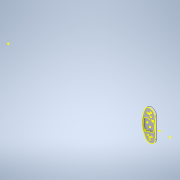
# Autodesk Inventor part: クランク
Saved by Autodesk Inventor 2022.2 (Build 262287000, 287)
## iProperties
Created: 2021-12-23
Part Number: クランク
Material: Generic
Document SubType Name: Modeling
Designer: acps
Density: 1 g/cm^3
Appearance: Default
Author: acps
Autodesk Inventor part; units mm, degrees
ref_plane "YZ Plane" through (0, 0, 0) normal (1, 0, 0) x (0, 1, 0)
ref_plane "XZ Plane" through (0, 0, 0) normal (0, 1, 0) x (-1, 0, 0)
ref_plane "XY Plane" through (0, 0, 0) normal (0, 0, 1) x (1, 0, 0)
sketch "Sketch1" plane through (0, 0, 0) normal (0, 0, 1) x (1, 0, 0)
  line L0 (-15.8764, 0) -> (-29.8764, 0)
  line L1 (-15.8764, 0) -> (-7.3764, 0)
  line L2 (-25.9706, 16.9706) -> (-25.9706, -16.9706) construction
  line L3 (-7.9706, -16.9706) -> (-7.9706, 16.9706) construction
  arc A0 (-7.9706, 16.9706) -> (-7.9926, 17.6) centre (-16.9706, 16.9706) ccw construction
  arc A1 (-25.9706, -16.9706) -> (-25.0651, -20.9049) centre (-16.9706, -16.9706) ccw construction
  arc A2 (-25.0651, 20.9049) -> (-25.0651, -20.9049) centre (17.9444, 0) ccw
  arc A3 (-7.9926, -17.6) -> (-7.9926, 17.6) centre (-259.0334, 0) ccw
  arc A4 (-25.0651, 20.9049) -> (-25.9706, 16.9706) centre (-16.9706, 16.9706) ccw construction
  arc A5 (-25.0651, -20.9049) -> (-7.9926, -17.6) centre (-16.9706, -16.9706) ccw
  arc A6 (-7.9926, 17.6) -> (-25.0651, 20.9049) centre (-16.9706, 16.9706) ccw
  arc A7 (-7.9926, -17.6) -> (-7.9706, -16.9706) centre (-16.9706, -16.9706) ccw construction
  line L4 (-16.9706, -20.5501) -> (-20.0706, -15.1808) construction
  line L5 (-20.0706, -15.1808) -> (-13.8706, -15.1808) construction
  line L6 (-13.8706, -15.1808) -> (-16.9706, -20.5501) construction
  circle A8 centre (-20.0706, -15.1808) radius 1.25
  circle A9 centre (-13.8706, -15.1808) radius 1.25
  circle A10 centre (-16.9706, -20.5501) radius 1.25
  line L7 (0, 0) -> (-43.2466, 0) construction
  line L8 (-15.1808, 20.0706) -> (-15.1808, 13.8706) construction
  line L9 (-15.1808, 13.8706) -> (-20.5501, 16.9706) construction
  line L10 (-20.5501, 16.9706) -> (-15.1808, 20.0706) construction
  circle A11 centre (-15.1808, 13.8706) radius 1.25
  circle A12 centre (-20.5501, 16.9706) radius 1.25
  circle A13 centre (-15.1808, 20.0706) radius 1.25
  line L11 (-16.9706, 16.9706) -> (0, 0) construction
  line L12 (-16.9706, -16.9706) -> (0, 0) construction
  point P0 (-29.8764, 0)
  point P1 (-7.3764, 0)
  dimension "d11" = 9
  dimension "d14" = 2.5
  dimension "d15" = 2.5
  dimension "d16" = 2.5
  dimension "d17" = 6.2
  dimension "d19" = 2.5
  dimension "d20" = 2.5
  dimension "d21" = 2.5
  dimension "d22" = 6.2
  dimension "d23" = 24
  dimension "d24" = 45
  dimension "d25" = 24
  dimension "d26" = 45
  dimension "d27" = 14
  dimension "d28" = 8.5
  constraints: 24 end point, 22 point on circle, 14 centre point, 8 coincident, 8 tangent, 4 horizontal, 2 point on line, 2 vertical, 24 other
  measures "d11" radius of A1
  measures "d14" diameter of A8
  measures "d15" diameter of A9
  measures "d16" diameter of A10
  measures "d17" distance of L5.end L4.end
  measures "d19" diameter of A11
  measures "d20" diameter of A12
  measures "d21" diameter of A13
  measures "d22" distance of L9.end L8.end
  measures "d23" distance of L11.start L7.start
  measures "d24" angle of L7 L11
  measures "d25" distance of L12.start L7.start
  measures "d26" angle of L7 L12
  measures "d27" distance of point (-29.876, 0) L0.start
  measures "d28" distance of point (-7.376, 0) L0.start
extrude "Extrusion1" add sketch "Sketch1" along normal blind 3
sketch "Sketch2" plane through (0, 0, 3) normal (0, 0, 1) x (1, 0, 0)
  arc A0 (-25.0651, 20.9049) -> (-25.0651, -20.9049) centre (17.9444, 0) ccw projected
  arc A1 (-25.0651, -20.9049) -> (-7.9926, -17.6) centre (-16.9706, -16.9706) ccw projected
  arc A2 (-7.9926, -17.6) -> (-7.9926, 17.6) centre (-259.0334, 0) ccw projected
  arc A3 (-7.9926, 17.6) -> (-25.0651, 20.9049) centre (-16.9706, 16.9706) ccw projected
  circle A4 centre (-16.9706, -20.5501) radius 1.25 projected
  circle A5 centre (-13.8706, -15.1808) radius 1.25 projected
  circle A6 centre (-20.0706, -15.1808) radius 1.25 projected
  circle A7 centre (-15.1808, 13.8706) radius 1.25 projected
  circle A8 centre (-15.1808, 20.0706) radius 1.25 projected
  circle A9 centre (-20.5501, 16.9706) radius 1.25 projected
  arc A10 (-23.2663, 20.0306) -> (-23.2663, -20.0306) centre (17.9444, 0) ccw
  arc A11 (-9.9877, 17.4601) -> (-23.2663, 20.0306) centre (-16.9706, 16.9706) ccw
  arc A12 (-9.9877, -17.4601) -> (-9.9877, 17.4601) centre (-259.0334, 0) ccw
  arc A13 (-23.2663, -20.0306) -> (-9.9877, -17.4601) centre (-16.9706, -16.9706) ccw
  circle A14 centre (-15.1808, 13.8706) radius 4.25
  circle A15 centre (-16.9706, 16.9706) radius 7.8296
  circle A16 centre (-16.9706, -16.9706) radius 7.8296
  line L0 (-9.7642, 13.9095) -> (10.6825, 13.9095)
  point P0 (0, 0)
  point P1 (-24.7881, -16.5371)
  point P2 (-9.7642, -13.9095)
  point P3 (-24.7881, 16.5371)
  dimension "d33" = 15.6591
  dimension "d31" = 2
  dimension "d32" = 3
  dimension "d34" = 15.6591
  constraints: 9 point on circle, 6 centre point, 2 coincident, 2 end point, 1 horizontal, 7 other
  measures "d31" radial gap between concentric circles of A0 A10
  measures "d32" radial gap between concentric circles of A7 A14
  measures "d34" diameter of A16
extrude "Extrusion2" cut sketch "Sketch2" against normal blind 2 contours A15 A12 A16 A10
fillet "Fillet1" radius 7 2 edges at (-24.7881, 16.5371, 2) (-9.7642, -13.9095, 2)
fillet "Fillet2" radius 2 2 edges at (-9.7642, 13.9095, 2) (-24.7881, -16.5371, 2)
sketch "Sketch3" plane through (0, 0, 3) normal (0, 0, 1) x (1, 0, 0)
  arc A0 (-18.9853, 9.4046) -> (-12.6387, 10.4485) centre (-16.9706, 16.9706) ccw projected
  arc A1 (-9.5334, 8.8534) -> (-12.6387, 10.4485) centre (-11.5322, 8.7825) ccw projected
  arc A2 (-9.3862, -2.2146) -> (-9.5334, 8.8534) centre (-259.0334, 0) ccw projected
  arc A3 (-16.6619, -9.1471) -> (-9.3862, -2.2146) centre (-16.386, -2.1525) ccw projected
  arc A4 (-16.6619, -9.1471) -> (-23.006, -11.983) centre (-16.9706, -16.9706) ccw projected
  arc A5 (-26.4871, -11.1978) -> (-23.006, -11.983) centre (-24.5477, -10.709) ccw projected
  arc A6 (-27.7703, 3.1165) -> (-26.4871, -11.1978) centre (17.9444, 0) ccw projected
  arc A7 (-18.9853, 9.4046) -> (-27.7703, 3.1165) centre (-20.7865, 2.6404) ccw projected
  arc A8 (-25.0651, 20.9049) -> (-25.0651, -20.9049) centre (17.9444, 0) ccw projected
  arc A9 (-25.0651, -20.9049) -> (-7.9926, -17.6) centre (-16.9706, -16.9706) ccw projected
  arc A10 (-7.9926, -17.6) -> (-7.9926, 17.6) centre (-259.0334, 0) ccw projected
  arc A11 (-7.9926, 17.6) -> (-25.0651, 20.9049) centre (-16.9706, 16.9706) ccw projected
  circle A12 centre (-16.9706, -20.5501) radius 1.25 projected
  circle A13 centre (-13.8706, -15.1808) radius 1.25 projected
  circle A14 centre (-20.0706, -15.1808) radius 1.25 projected
  circle A15 centre (-15.1808, 13.8706) radius 1.25 projected
  circle A16 centre (-15.1808, 20.0706) radius 1.25 projected
  circle A17 centre (-20.5501, 16.9706) radius 1.25 projected
  point P0 (0, 0)
equation "\"d34\" = d33"
body "Solid1"
